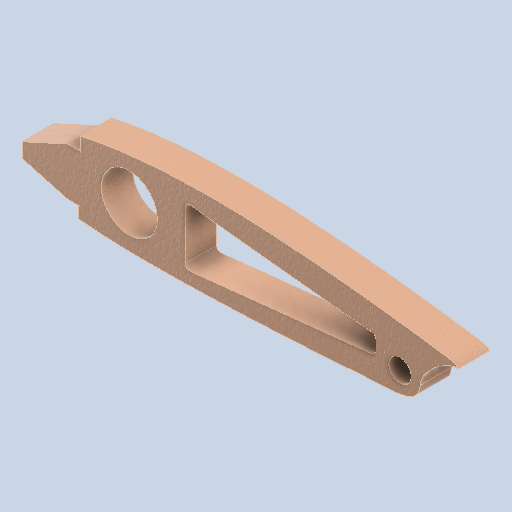
# Autodesk Inventor part: 3P.03.10.02.JS.rib 10 foam_CPY
Saved by Autodesk Inventor 2025.1 (Build 291241000, 241)
## iProperties
Created: 2025-01-11
Part Number: 3P.03.10.02.JS.rib 10 foam_CPY
Material: Generic
Document SubType Name: Modeling
Designer: johan
Density: 1 g/cm^3
Appearance: Default
Author: thoma
Autodesk Inventor part; units mm, degrees
ref_plane "YZ Plane" through (0, 0, 0) normal (1, 0, 0) x (0, 1, 0)
ref_plane "XZ Plane" through (0, 0, 0) normal (0, 1, 0) x (-1, 0, 0)
ref_plane "XY Plane" through (0, 0, 0) normal (0, 0, 1) x (1, 0, 0)
sketch "Sketch3" plane through (0, 0, 0) normal (0, 0, 1) x (1, 0, 0)
  line L0 (-80.5781, 0.8246) -> (-80.5781, 20.7988) construction
  circle A0 centre (-80.5781, 0.8246) radius 13.481
  line L1 (-53.718, 12.5571) -> (-53.718, -10.9927)
  arc A1 (-53.718, -10.9927) -> (-51.5055, -12.9814) centre (-51.718, -10.9927) ccw
  arc A2 (-51.5055, 14.5458) -> (-53.718, 12.5571) centre (-51.718, 12.5571) ccw
  line L2 (36.2228, -3.6088) -> (-51.5055, -12.9814)
  line L3 (38.0103, 3.1845) -> (38.0103, -1.6201)
  line L4 (-80.5781, 0.8246) -> (49.5525, 0.8246) construction
  circle A3 centre (49.6953, -3.8247) radius 5.3555
  line L5 (59.6953, 14.884) -> (59.6953, -12.7998) construction
  spline S0 degree 4 poles (77.9414, 11.0338) (75.5683, 12.9654) (71.7145, 13.0272) (66.8099, 13.9036) (60.7685, 14.7338) (56.2959, 15.3578) (51.7728, 15.9509) (47.2242, 16.5426) (42.6244, 17.1111) (37.9974, 17.6651) (33.3378, 18.1987) (28.6546, 18.7114) (23.9504, 19.2026) (19.2309, 19.6699) (14.5002, 20.1135) (9.7632, 20.5291) (5.025, 20.9191) (0.2903, 21.2792) (-4.4372, 21.6095) (-9.151, 21.9092) (-13.8524, 22.1766) (-18.5268, 22.4102) (-23.2002, 22.6105) (-27.8558, 22.7627) (-32.4748, 22.8704) (-37.0553, 22.9312) (-41.5904, 22.9454) (-46.0738, 22.9127) (-50.5027, 22.8323) (-54.8678, 22.7052) (-59.1755, 22.5324) (-63.394, 22.3084) (-67.5752, 22.0492) (-71.5451, 21.7209) (-75.7777, 21.4072) (-79.04, 20.9063) (-83.4863, 20.5541) (-87.0067, 20.037) (-90.7113, 19.5168) (-94.2172, 18.9459) (-97.6363, 18.3426) (-100.9342, 17.7015) (-104.1216, 17.0263) (-107.1909, 16.3187) (-110.1396, 15.5797) (-112.9656, 14.8117) (-115.6652, 14.0172) (-118.2357, 13.1965) (-120.6759, 12.3541) (-122.9817, 11.4895) (-125.1529, 10.6071) (-127.1857, 9.7065) (-129.0794, 8.7914) (-130.8324, 7.8633) (-132.4429, 6.923) (-133.9096, 5.9737) (-135.2322, 5.016) (-136.4083, 4.0508) (-137.4392, 3.0816) (-138.3215, 2.1025) (-139.0592, 1.1321) (-139.6407, 0.1249) (-140.106, -0.8362) (-140.3589, -2.0477) (-140.602, -2.598) (-140.1166, -5.4607) (-140.0539, -5.4622) (-139.4639, -6.7645) (-138.8842, -7.4979) (-138.1173, -8.3934) (-137.2199, -9.1877) (-136.1721, -9.9852) (-134.9893, -10.738) (-133.6669, -11.4655) (-132.2091, -12.1599) (-130.6156, -12.8245) (-128.8897, -13.4579) (-127.0312, -14.0591) (-125.0439, -14.6296) (-122.9287, -15.1678) (-120.6879, -15.6738) (-118.3241, -16.1476) (-115.8396, -16.5892) (-113.2366, -16.9984) (-110.5176, -17.3742) (-107.6861, -17.7183) (-104.7439, -18.0297) (-101.6943, -18.3095) (-98.5398, -18.5568) (-95.2843, -18.7732) (-91.9297, -18.9579) (-88.48, -19.1131) (-84.9381, -19.2376) (-81.3071, -19.3341) (-77.5906, -19.4015) (-73.7915, -19.4421) (-69.9139, -19.4561) (-65.961, -19.445) (-61.9362, -19.4102) (-57.8434, -19.3518) (-53.6861, -19.2727) (-49.4679, -19.1731) (-45.1932, -19.0538) (-40.8649, -18.9183) (-36.4879, -18.766) (-32.0649, -18.5992) (-27.598, -18.4192) (-23.0941, -18.227) (-18.5434, -18.0273) (-13.9382, -17.8076) (-9.3141, -17.5719) (-4.666, -17.3195) (-0.0002, -17.052) (4.6675, -16.7728) (9.3655, -16.4759) (14.0236, -16.1832) (19.545, -15.7815) (23.3079, -15.6072) (27.1098, -15.1781) (28.8959, -15.0599) knots 0 0 0 0 0 0.024672 0.034555 0.0445 0.054495 0.064543 0.074632 0.084755 0.094911 0.105094 0.115299 0.125521 0.135755 0.145995 0.156237 0.166475 0.176705 0.186921 0.197118 0.207299 0.217463 0.227605 0.23772 0.247796 0.257824 0.267798 0.277713 0.287563 0.297345 0.307053 0.31668 0.326224 0.335555 0.344908 0.354162 0.363308 0.372467 0.381393 0.390196 0.398872 0.407415 0.41582 0.424082 0.432193 0.44015 0.447945 0.455574 0.46303 0.470307 0.477401 0.484305 0.491015 0.497525 0.503831 0.509931 0.515822 0.521506 0.526986 0.53227 0.537373 0.542316 0.547131 0.552525 0.557529 0.562533 0.567581 0.57205 0.576988 0.582082 0.587354 0.592817 0.598478 0.604341 0.610406 0.616671 0.623133 0.629789 0.636632 0.643658 0.650861 0.658236 0.665777 0.673478 0.681333 0.689338 0.697486 0.705771 0.71419 0.722736 0.731403 0.740188 0.749084 0.758087 0.767192 0.776393 0.785687 0.795067 0.804529 0.814069 0.823682 0.833362 0.843106 0.852907 0.862763 0.872667 0.88262 0.892624 0.902675 0.912766 0.92289 0.933033 0.943191 0.953358 0.963531 0.973703 0.984092 1 1 1 1 1
  line L6 (7.5013, -16.4763) -> (50.2906, -13.6435) construction
  arc A4 (44.8353, -17.2546) -> (13.385, -19.3367) centre (31.5327, -54.8885) ccw construction
  line L7 (159.6953, -3.8066) -> (59.6953, -3.8066) construction
  line L8 (-51.5055, 14.5458) -> (36.2228, 5.1732)
  arc A5 (36.2228, -3.6088) -> (38.0103, -1.6201) centre (36.0103, -1.6201) ccw
  arc A6 (38.0103, 3.1845) -> (36.2228, 5.1732) centre (36.0103, 3.1845) ccw
  spline S1 degree 4 poles (78.1029, 11.0141) (76.6463, 11.2227) (73.9909, 10.5042) (70.2765, 8.6041) (66.0429, 5.3938) (62.3889, 1.8499) (60.314, -1.2467) (59.5572, -3.5763) (59.5773, -5.0793) knots 0 0 0 0 0 0.302475 0.43895 0.576633 0.708802 1 1 1 1 1
  spline S2 degree 4 poles (28.8959, -15.0599) (34.0984, -14.7105) (49.269, -14.182) (58.5645, -15.239) (59.5773, -5.0793) knots 0 0 0 0 0 1 1 1 1 1
  line L9 (28.8959, -15.0599) -> (34.0984, -14.7105) construction
  line L10 (34.0984, -14.7105) -> (49.269, -14.182) construction
  line L11 (49.269, -14.182) -> (58.5645, -15.239) construction
  line L12 (58.5645, -15.239) -> (59.5773, -5.0793) construction
  line L13 (-140.4646, -2.8394) -> (159.4818, -3.8173) construction
  line L14 (-132.0856, 0.6333) -> (-132.0856, -6.3667)
  line L15 (-132.0856, -6.3667) -> (-110.3816, -12.3574)
  line L16 (-110.3816, -12.3574) -> (-104.797, -12.3574)
  line L17 (-104.797, -12.3574) -> (-104.797, -18.0156)
  line L18 (-132.0856, 0.6333) -> (-110.3816, 10.553)
  line L19 (-110.3816, 10.553) -> (-104.1736, 10.553)
  line L20 (-104.1736, 10.553) -> (-104.1736, 17.0026)
  point P0 (0, 0)
  point P1 (17.6589, 23.5628)
  point P2 (75.883, 10.8572)
  point P3 (72.8647, 9.7686)
  point P4 (69.4179, 7.8149)
  point P5 (66.0452, 5.2617)
  point P6 (63.1887, 2.4463)
  point P7 (61.1228, -0.3317)
  point P8 (59.9357, -2.8689)
  point P9 (-160.0931, -3.8671)
  point P10 (28.8959, -15.0599)
  point P11 (69.5533, 13.4647)
  point P12 (65.1899, 14.1023)
  point P13 (60.7936, 14.7318)
  point P14 (56.3207, 15.3468)
  point P15 (51.7945, 15.947)
  point P16 (47.2398, 16.5346)
  point P17 (42.6414, 17.1053)
  point P18 (38.0104, 17.6585)
  point P19 (33.3491, 18.1925)
  point P20 (28.6632, 18.7055)
  point P21 (23.9568, 19.1966)
  point P22 (19.2348, 19.6643)
  point P23 (14.5017, 20.1074)
  point P24 (9.7623, 20.5238)
  point P25 (5.0217, 20.9132)
  point P26 (0.2844, 21.2735)
  point P27 (-4.4451, 21.6038)
  point P28 (-9.1614, 21.9032)
  point P29 (-13.86, 22.1702)
  point P30 (-18.5361, 22.4036)
  point P31 (-23.211, 22.601)
  point P32 (-27.8721, 22.754)
  point P33 (-32.4966, 22.8611)
  point P34 (-37.0797, 22.9217)
  point P35 (-41.6169, 22.9356)
  point P36 (-46.1028, 22.9023)
  point P37 (-50.5329, 22.8216)
  point P38 (-54.9021, 22.6941)
  point P39 (-59.2065, 22.5195)
  point P40 (-63.4406, 22.2977)
  point P41 (-67.6008, 22.0302)
  point P42 (-71.6806, 21.7165)
  point P43 (-75.6814, 21.3591)
  point P44 (-79.1834, 20.9458)
  point P45 (-83.4048, 20.5095)
  point P46 (-87.1309, 20.023)
  point P47 (-90.7527, 19.494)
  point P48 (-94.2725, 18.9266)
  point P49 (-97.6845, 18.3211)
  point P50 (-100.9861, 17.6791)
  point P51 (-107.2438, 16.2934)
  point P52 (-110.1931, 15.553)
  point P53 (-113.0194, 14.7835)
  point P54 (-115.7191, 13.987)
  point P55 (-118.2898, 13.165)
  point P56 (-120.7294, 12.3201)
  point P57 (-123.0349, 11.454)
  point P58 (-125.2048, 10.569)
  point P59 (-127.2364, 9.6666)
  point P60 (-129.1282, 8.7491)
  point P61 (-130.8786, 7.8185)
  point P62 (-132.486, 6.8762)
  point P63 (-133.9488, 5.9245)
  point P64 (-135.2661, 4.9648)
  point P65 (-136.4363, 3.9987)
  point P66 (-137.4592, 3.0275)
  point P67 (-138.3336, 2.0531)
  point P68 (-139.0591, 1.0763)
  point P69 (-139.6352, 0.0983)
  point P70 (-140.0613, -0.8802)
  point P71 (-140.338, -1.8576)
  point P72 (-140.1239, -5.2398)
  point P73 (-139.9547, -5.7022)
  point P74 (-139.492, -6.6066)
  point P75 (-138.8844, -7.4823)
  point P76 (-138.1328, -8.3292)
  point P77 (-137.2384, -9.147)
  point P78 (-136.202, -9.9355)
  point P79 (-135.0249, -10.6943)
  point P80 (-133.7085, -11.4228)
  point P81 (-132.2548, -12.1206)
  point P82 (-130.6648, -12.7879)
  point P83 (-128.941, -13.4239)
  point P84 (-127.0846, -14.0282)
  point P85 (-125.0983, -14.6009)
  point P86 (-122.9839, -15.1415)
  point P87 (-120.7435, -15.6497)
  point P88 (-118.3798, -16.1256)
  point P89 (-115.8952, -16.569)
  point P90 (-113.2918, -16.9797)
  point P91 (-110.5723, -17.3574)
  point P92 (-107.74, -17.7027)
  point P93 (-101.7463, -18.2964)
  point P94 (-98.5909, -18.5451)
  point P95 (-95.3341, -18.7623)
  point P96 (-91.9783, -18.9484)
  point P97 (-88.5271, -19.1041)
  point P98 (-84.9838, -19.2298)
  point P99 (-81.3514, -19.3267)
  point P100 (-77.6332, -19.3951)
  point P101 (-73.8324, -19.4362)
  point P102 (-69.9531, -19.4509)
  point P103 (-65.9985, -19.4404)
  point P104 (-61.9719, -19.4059)
  point P105 (-57.8772, -19.3483)
  point P106 (-53.718, -19.2694)
  point P107 (-49.4979, -19.1701)
  point P108 (-45.2211, -19.0516)
  point P109 (-40.8909, -18.916)
  point P110 (-36.5118, -18.7642)
  point P111 (-32.0871, -18.5977)
  point P112 (-27.6213, -18.418)
  point P113 (-23.1183, -18.2269)
  point P114 (-18.5646, -18.0247)
  point P115 (-13.9566, -17.8054)
  point P116 (-9.3252, -17.5693)
  point P117 (-4.674, -17.317)
  point P118 (-0.0078, -17.05)
  point P119 (4.6686, -16.7695)
  point P120 (9.3513, -16.477)
  point P121 (14.0352, -16.1731)
  point P122 (18.7161, -15.8596)
  point P123 (23.3889, -15.5371)
  point P124 (78.0825, 12.164)
  point P125 (159.2574, -3.8401)
  point P126 (158.8836, -3.8779)
  point P127 (158.3607, -3.9307)
  point P128 (157.6896, -3.9985)
  point P129 (156.8706, -4.081)
  point P130 (155.9046, -4.1779)
  point P131 (154.7931, -4.2892)
  point P132 (153.5367, -4.4143)
  point P133 (152.1372, -4.5532)
  point P134 (150.5955, -4.7056)
  point P135 (148.914, -4.8712)
  point P136 (147.0936, -5.0494)
  point P137 (145.137, -5.2399)
  point P138 (143.0457, -5.4421)
  point P139 (140.8221, -5.6563)
  point P140 (138.4686, -5.8813)
  point P141 (135.9876, -6.1174)
  point P142 (133.3815, -6.3634)
  point P143 (130.6533, -6.6196)
  point P144 (127.8054, -6.8851)
  point P145 (124.8414, -7.1596)
  point P146 (121.7634, -7.4428)
  point P147 (118.5756, -7.7341)
  point P148 (115.2804, -8.0332)
  point P149 (111.8817, -8.3395)
  point P150 (108.3828, -8.6527)
  point P151 (104.787, -8.9722)
  point P152 (101.0985, -9.2974)
  point P153 (97.3206, -9.6283)
  point P154 (93.4572, -9.9643)
  point P155 (89.5122, -10.3048)
  point P156 (85.4898, -10.6492)
  point P157 (81.3936, -10.9969)
  point P158 (77.2284, -11.3479)
  point P159 (72.9975, -11.701)
  point P160 (68.7057, -12.0556)
  point P161 (64.3572, -12.4117)
  point P162 (59.9559, -12.7678)
  point P163 (55.5069, -13.1239)
  point P164 (51.0138, -13.4788)
  point P165 (46.4817, -13.8316)
  point P166 (41.9148, -14.182)
  point P167 (35.7035, -14.3277)
  point P168 (32.6946, -14.8708)
  point P169 (82.2459, 11.5043)
  point P170 (86.3364, 10.8401)
  point P171 (90.3495, 10.1732)
  point P172 (94.2816, 9.5051)
  point P173 (98.1288, 8.837)
  point P174 (101.8872, 8.171)
  point P175 (105.5538, 7.5086)
  point P176 (109.1244, 6.8507)
  point P177 (112.596, 6.1997)
  point P178 (115.9653, 5.5565)
  point P179 (119.2287, 4.9229)
  point P180 (122.3835, 4.3007)
  point P181 (125.4264, 3.6911)
  point P182 (128.3547, 3.0956)
  point P183 (131.1654, 2.5157)
  point P184 (133.8561, 1.9532)
  point P185 (136.4244, 1.4093)
  point P186 (138.8676, 0.8855)
  point P187 (141.1833, 0.383)
  point P188 (143.3697, -0.0964)
  point P189 (145.4247, -0.5518)
  point P190 (147.3462, -0.9817)
  point P191 (149.1327, -1.3852)
  point P192 (150.7821, -1.7608)
  point P193 (152.2935, -2.1073)
  point P194 (153.6651, -2.4241)
  point P195 (154.8954, -2.7103)
  point P196 (155.9838, -2.9647)
  point P197 (156.9291, -3.187)
  point P198 (157.7307, -3.376)
  point P199 (158.3871, -3.5317)
  dimension "d3" = 26.962
  dimension "d6" = 10.711
  dimension "d7" = 110
  dimension "d8" = 100
  dimension "d9" = 2
  dimension "d11" = 4.6493
  dimension "d25" = 7
  dimension "d26" = 3.5
  dimension "d27" = 8.379
  dimension "d28" = 30.083
  dimension "d29" = 5
  dimension "d30" = 5
  dimension "d31" = 59.8865
  constraints: 34 end point, 11 point on circle, 8 tangent, 7 centre point, 5 vertical, 3 equal radius, 3 horizontal, 3 midpoint, 3 perpendicular, 1 point on line, 138 other
  measures "d3" diameter of A0
  measures "d6" diameter of A3
  measures "d7" distance of L7.start A3.centre
  measures "d8" distance of L7.start L7.end
  measures "d9" radius of A2
  measures "d11" vertical distance of A3.centre L0.start
  measures "d25" distance of L14.end L14.start
  measures "d26" distance from line of L13 L14.start
  measures "d27" horizontal distance of point (-132.086, -2.867) L13.start
  measures "d28" horizontal distance of L15.end L13.start
  measures "d29" vertical distance of point (-110.193, 15.553) L18.end
  measures "d30" vertical distance of point (-110.572, -17.357) L15.end
  measures "d31" horizontal distance of L13.start L0.start
extrude "Extrusion2" add sketch "Sketch3" along normal blind 15 contours S1 S2 S0 L17 L16 L15 L14 L18 L19 L20
body "Solid2"
